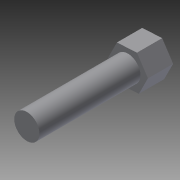
# Autodesk Inventor part: nut
Saved by Autodesk Inventor 2013 (Build 170138000, 138)
## iProperties
Created: 2015-09-10
Part Number: nut
Material: Generic
Document SubType Name: Modeling
Designer: Students
Density: 1 g/cm^3
Author: Students
Autodesk Inventor part; units mm, degrees
ref_plane "YZ Plane" through (0, 0, 0) normal (1, 0, 0) x (0, 1, 0)
ref_plane "XZ Plane" through (0, 0, 0) normal (0, 1, 0) x (-1, 0, 0)
ref_plane "XY Plane" through (0, 0, 0) normal (0, 0, 1) x (1, 0, 0)
sketch "Sketch1" plane through (0, 0, 0) normal (0, 1, 0) x (-1, 0, 0)
  circle A0 centre (0, 0) radius 2.5
  dimension "d0" = 5
  constraints: 1 centre point, 1 coincident
  measures "d0" diameter of A0
extrude "Extrusion1" add sketch "Sketch1" along normal blind 20
sketch "Sketch2" plane through (0, 20, 0) normal (0, 1, 0) x (1, 0, 0)
  circle A0 centre (0, 0) radius 2.5 projected
  line L0 (1.7855, -3.5367) -> (-2.1701, -3.3146)
  line L1 (-2.1701, -3.3146) -> (-3.9556, 0.222)
  line L2 (-3.9556, 0.222) -> (-1.7855, 3.5367)
  line L3 (-1.7855, 3.5367) -> (2.1701, 3.3146)
  line L4 (2.1701, 3.3146) -> (3.9556, -0.222)
  line L5 (3.9556, -0.222) -> (1.7855, -3.5367)
  constraints: 12 end point, 1 coincident, 13 other
extrude "Extrusion2" add sketch "Sketch2" along normal blind 5
body "Solid1"
